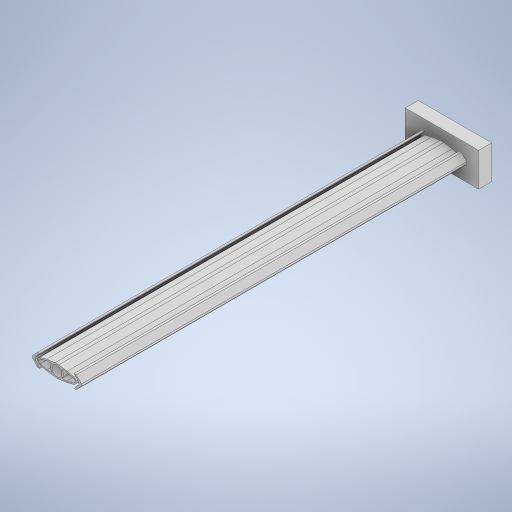
# Autodesk Inventor part: Enemy_gun_inertia_modell
Saved by Autodesk Inventor 2024 (Build 280153000, 153)
## iProperties
Created: 2026-05-20
Part Number: Enemy_gun_inertia_modell
Material: Generic
Document SubType Name: Modeling
Designer: warny
Mass: 606.653 g
Surface Area: 3403.99 cm^2
Volume: 606.653 cm^3
Density: 1 g/cm^3
Appearance: Default
Author: warny
Autodesk Inventor part; units mm, degrees
ref_plane "YZ Plane" through (0, 0, 0) normal (1, 0, 0) x (0, 1, 0)
ref_plane "XZ Plane" through (0, 0, 0) normal (0, 1, 0) x (-1, 0, 0)
ref_plane "XY Plane" through (0, 0, 0) normal (0, 0, 1) x (1, 0, 0)
sketch "Sketch1" plane through (0, 0, 0) normal (0, 0, 1) x (1, 0, 0)
  line L0 (0, -41.16) -> (0, 41.16) projected
  line L1 (-89.6, 0) -> (89.6, 0) projected
  line L2 (0, 11.3) -> (18, 8.7)
  line L3 (18, 8.7) -> (30, 5.7)
  line L4 (30, 5.7) -> (34, 1.7)
  line L5 (34, 1.7) -> (34, 0)
  line L6 (0, 6.6) -> (17, 6.6)
  line L7 (17, 6.6) -> (29, 3.6)
  line L8 (29, 3.6) -> (32, 0.9)
  line L9 (32, 0.9) -> (32, 0)
  line L10 (38, 0) -> (38, 1.7)
  line L11 (38, 1.7) -> (30, 11.3)
  line L12 (30, 11.3) -> (34, 11.3)
  line L13 (34, 11.3) -> (43, 1.7)
  line L14 (43, 1.7) -> (43, 0)
  line L15 (-64, -29.4) -> (64, -29.4)
  line L16 (64, -29.4) -> (64, 29.4)
  line L17 (64, 29.4) -> (-64, 29.4)
  line L18 (-64, 29.4) -> (-64, -29.4)
  line L19 (-64, -29.4) -> (64, 29.4) construction
  line L20 (64, -29.4) -> (-64, 29.4) construction
  point P0 (0, 0)
  dimension "d1" = 18
  dimension "d2" = 30
  dimension "d3" = 34
  dimension "d5" = 5.7
  dimension "d6" = 1.7
  dimension "d7" = 6.6
  dimension "d8" = 3.6
  dimension "d9" = 0.9
  dimension "d10" = 17
  dimension "d11" = 29
  dimension "d12" = 32
  dimension "d13" = 8.7
  dimension "d14" = 11.3
  dimension "d20" = 11.3
  dimension "d21" = 30
  dimension "d22" = 34
  dimension "d23" = 38
  dimension "d24" = 43
  dimension "d25" = 1.7
  dimension "d26" = 1.7
  dimension "d27" = 29.4
  dimension "d28" = 64
  constraints: 38 end point, 6 point on line, 5 perpendicular, 2 midpoint, 2 parallel, 2 vertical, 1 horizontal
  measures "d1" distance from line of L2.end L0
  measures "d2" distance from line of L0 L3.end
  measures "d3" distance from line of L0 L4.end
  measures "d5" distance from line of L1 L3.end
  measures "d6" distance from line of L1 L4.end
  measures "d7" distance of point (0, 0) L6.start
  measures "d8" distance from line of L1 L7.end
  measures "d9" distance from line of L1 L8.end
  measures "d10" distance from line of L0 L6.end
  measures "d11" distance from line of L0 L7.end
  measures "d12" distance from line of L0 L8.end
  measures "d13" distance from line of L1 L2.end
  measures "d14" distance from line of L1 L2.start
  measures "d20" distance between parallel lines of L1 L12
  measures "d21" distance from line of L0 L11.end
  measures "d22" distance from line of L0 L12.end
  measures "d23" distance from line of L0 L10.end
  measures "d24" distance from line of L0 L13.end
  measures "d25" distance from line of L1 L10.end
  measures "d26" distance from line of L1 L13.end
  measures "d27" distance from line of L1 L16.end
  measures "d28" distance between parallel lines of L18 L0
extrude "Extrusion1" add sketch "Sketch1" along normal blind 672.2 contours L0 L2 L3 L4 L5 L1 L9 L8 L7 L6 | L10 L11 L12 L13 L14 L1
mirror "Mirror1" about plane through (0, 0, 0) normal (1, 0, 0) of "Extrusion1"
mirror "Mirror2" about plane through (0, 0, 0) normal (0, 1, 0) of "Extrusion1", "Mirror1"
extrude "Extrusion2" add sketch "Sketch1" against normal blind 22.8 contours L0 L1 L18 L17 | L6 L7 L8 L9 L1 L0 | L0 L17 L16 L1 L14 L13 L12 L11 L10 L5 L4 L3 L2 | L1 L16 L15 L0 | L0 L15 L18 L1
sketch "Sketch2" plane through (0, 0, 672.2) normal (0, 0, 1) x (1, 0, 0)
  circle A0 centre (0, 0) radius 11.3
  dimension "d33" = 22.6
  constraints: 1 centre point, 1 coincident
  measures "d33" diameter of A0
extrude "Extrusion3" add sketch "Sketch2" against normal up to next
sketch "Sketch3" plane through (0, 0, 672.2) normal (0, 0, 1) x (1, 0, 0)
  circle A0 centre (0, 0) radius 8.6
  dimension "d36" = 17.2
  constraints: 1 centre point, 1 coincident
  measures "d36" diameter of A0
extrude "Extrusion4" cut sketch "Sketch3" against normal through all
body "Solid1"
